Autodesk Fusion 360 part; units mm, degrees
(part 2 of 3)
  spline S18 degree 5 poles (2.4575, 16.735) (2.4592, 16.7471) (2.4624, 16.7712) (2.466, 16.8075) (2.4685, 16.8561) (2.4687, 16.9171) (2.4667, 16.9782) (2.4633, 17.0395) (2.4593, 17.1009) (2.4548, 17.1623) (2.4497, 17.2237) (2.4439, 17.2852) (2.4372, 17.3467) (2.4294, 17.4083) (2.4206, 17.4699) (2.4107, 17.5316) (2.4, 17.5933) (2.3886, 17.6549) (2.3766, 17.7166) (2.364, 17.7783) (2.3508, 17.84) (2.337, 17.9017) (2.3225, 17.9634) (2.3073, 18.025) (2.2914, 18.0867) (2.2749, 18.1483) (2.2578, 18.2099) (2.2401, 18.2715) (2.2219, 18.3331) (2.2031, 18.3946) (2.1837, 18.4561) (2.1638, 18.5175) (2.1433, 18.579) (2.1223, 18.6403) (2.1007, 18.7017) (2.0786, 18.763) (2.056, 18.8242) (2.0329, 18.8854) (2.0092, 18.9465) (1.9851, 19.0076) (1.9605, 19.0686) (1.9353, 19.1296) (1.9097, 19.1905) (1.8836, 19.2514) (1.857, 19.3121) (1.8299, 19.3728) (1.8024, 19.4335) (1.7743, 19.494) (1.7459, 19.5545) (1.7169, 19.615) (1.6875, 19.6753) (1.6577, 19.7355) (1.6274, 19.7957) (1.5966, 19.8558) (1.5654, 19.9158) (1.5338, 19.9757) (1.5017, 20.0356) (1.4692, 20.0953) (1.4362, 20.155) (1.4029, 20.2145) (1.3691, 20.274) (1.3348, 20.3333) (1.3002, 20.3926) (1.2651, 20.4518) (1.2296, 20.5108) (1.1937, 20.5698) (1.1574, 20.6286) (1.1207, 20.6874) (1.0836, 20.746) (1.0461, 20.8045) (1.0082, 20.8629) (0.9775, 20.9095) (0.9544, 20.9445) (0.9388, 20.9677) (0.931, 20.9794) knots 0 0 0 0 0 0 0.01428571 0.02857143 0.04285714 0.05714286 0.07142857 0.08571429 0.1 0.11428571 0.12857143 0.14285714 0.15714286 0.17142857 0.18571429 0.2 0.21428571 0.22857143 0.24285714 0.25714286 0.27142857 0.28571429 0.3 0.31428571 0.32857143 0.34285714 0.35714286 0.37142857 0.38571429 0.4 0.41428571 0.42857143 0.44285714 0.45714286 0.47142857 0.48571429 0.5 0.51428571 0.52857143 0.54285714 0.55714286 0.57142857 0.58571429 0.6 0.61428571 0.62857143 0.64285714 0.65714286 0.67142857 0.68571429 0.7 0.71428571 0.72857143 0.74285714 0.75714286 0.77142857 0.78571429 0.8 0.81428571 0.82857143 0.84285714 0.85714286 0.87142857 0.88571429 0.9 0.91428571 0.92857143 0.94285714 0.95714286 0.97142857 0.98571429 1 1 1 1 1 1
  arc A29 (0.931, 20.9794) -> (-0.931, 20.9794) centre (0, 0) ccw
  spline S19 degree 5 poles (-0.931, 20.9794) (-0.9388, 20.9677) (-0.9544, 20.9445) (-0.9775, 20.9095) (-1.0082, 20.8629) (-1.0461, 20.8045) (-1.0836, 20.746) (-1.1207, 20.6874) (-1.1574, 20.6286) (-1.1937, 20.5698) (-1.2296, 20.5108) (-1.2651, 20.4518) (-1.3002, 20.3926) (-1.3348, 20.3333) (-1.3691, 20.274) (-1.4029, 20.2145) (-1.4362, 20.155) (-1.4692, 20.0953) (-1.5017, 20.0356) (-1.5338, 19.9757) (-1.5654, 19.9158) (-1.5966, 19.8558) (-1.6274, 19.7957) (-1.6577, 19.7355) (-1.6875, 19.6753) (-1.7169, 19.615) (-1.7459, 19.5545) (-1.7743, 19.494) (-1.8024, 19.4335) (-1.8299, 19.3728) (-1.857, 19.3121) (-1.8836, 19.2514) (-1.9097, 19.1905) (-1.9353, 19.1296) (-1.9605, 19.0686) (-1.9851, 19.0076) (-2.0092, 18.9465) (-2.0329, 18.8854) (-2.056, 18.8242) (-2.0786, 18.763) (-2.1007, 18.7017) (-2.1223, 18.6403) (-2.1433, 18.579) (-2.1638, 18.5175) (-2.1837, 18.4561) (-2.2031, 18.3946) (-2.2219, 18.3331) (-2.2401, 18.2715) (-2.2578, 18.2099) (-2.2749, 18.1483) (-2.2914, 18.0867) (-2.3073, 18.025) (-2.3225, 17.9634) (-2.337, 17.9017) (-2.3508, 17.84) (-2.364, 17.7783) (-2.3766, 17.7166) (-2.3886, 17.6549) (-2.4, 17.5933) (-2.4107, 17.5316) (-2.4206, 17.4699) (-2.4294, 17.4083) (-2.4372, 17.3467) (-2.4439, 17.2852) (-2.4497, 17.2237) (-2.4548, 17.1623) (-2.4593, 17.1009) (-2.4633, 17.0395) (-2.4667, 16.9782) (-2.4687, 16.9171) (-2.4685, 16.8561) (-2.466, 16.8075) (-2.4624, 16.7712) (-2.4592, 16.7471) (-2.4575, 16.735) knots -1 -1 -1 -1 -1 -1 -0.98571429 -0.97142857 -0.95714286 -0.94285714 -0.92857143 -0.91428571 -0.9 -0.88571429 -0.87142857 -0.85714286 -0.84285714 -0.82857143 -0.81428571 -0.8 -0.78571429 -0.77142857 -0.75714286 -0.74285714 -0.72857143 -0.71428571 -0.7 -0.68571429 -0.67142857 -0.65714286 -0.64285714 -0.62857143 -0.61428571 -0.6 -0.58571429 -0.57142857 -0.55714286 -0.54285714 -0.52857143 -0.51428571 -0.5 -0.48571429 -0.47142857 -0.45714286 -0.44285714 -0.42857143 -0.41428571 -0.4 -0.38571429 -0.37142857 -0.35714286 -0.34285714 -0.32857143 -0.31428571 -0.3 -0.28571429 -0.27142857 -0.25714286 -0.24285714 -0.22857143 -0.21428571 -0.2 -0.18571429 -0.17142857 -0.15714286 -0.14285714 -0.12857143 -0.11428571 -0.1 -0.08571429 -0.07142857 -0.05714286 -0.04285714 -0.02857143 -0.01428571 0 0 0 0 0 0
  line L19 (-2.4575, 16.735) -> (-2.2515, 15.3323)
  arc A30 (-3.0322, 14.2091) -> (-2.2515, 15.3323) centre (-3.2409, 15.1871) ccw
  arc A31 (-5.7163, 14.4039) -> (-4.4786, 13.8215) centre (-4.7868, 14.7728) ccw
  line L20 (-5.7163, 14.4039) -> (-6.2393, 15.7217)
  spline S20 degree 5 poles (-6.2393, 15.7217) (-6.2438, 15.733) (-6.2531, 15.7555) (-6.2682, 15.7887) (-6.2903, 15.8321) (-6.3206, 15.885) (-6.3529, 15.9369) (-6.3864, 15.9883) (-6.4206, 16.0394) (-6.4553, 16.0903) (-6.4904, 16.141) (-6.5261, 16.1914) (-6.5627, 16.2413) (-6.6002, 16.2907) (-6.6387, 16.3397) (-6.678, 16.3882) (-6.7181, 16.4362) (-6.7588, 16.4839) (-6.8001, 16.5314) (-6.8418, 16.5785) (-6.8841, 16.6253) (-6.927, 16.6718) (-6.9703, 16.718) (-7.0143, 16.7638) (-7.0589, 16.8092) (-7.104, 16.8544) (-7.1496, 16.8992) (-7.1957, 16.9436) (-7.2423, 16.9878) (-7.2894, 17.0317) (-7.3369, 17.0753) (-7.3849, 17.1185) (-7.4333, 17.1615) (-7.4822, 17.2042) (-7.5315, 17.2465) (-7.5813, 17.2885) (-7.6315, 17.3303) (-7.6822, 17.3717) (-7.7332, 17.4128) (-7.7847, 17.4536) (-7.8365, 17.4942) (-7.8888, 17.5344) (-7.9414, 17.5743) (-7.9944, 17.614) (-8.0479, 17.6533) (-8.1017, 17.6923) (-8.1559, 17.7311) (-8.2104, 17.7695) (-8.2653, 17.8077) (-8.3206, 17.8455) (-8.3762, 17.8831) (-8.4322, 17.9203) (-8.4885, 17.9573) (-8.5452, 17.9939) (-8.6022, 18.0303) (-8.6596, 18.0664) (-8.7173, 18.1022) (-8.7753, 18.1376) (-8.8337, 18.1728) (-8.8924, 18.2077) (-8.9514, 18.2423) (-9.0107, 18.2766) (-9.0703, 18.3106) (-9.1303, 18.3443) (-9.1905, 18.3777) (-9.2511, 18.4108) (-9.3119, 18.4436) (-9.3731, 18.4761) (-9.4345, 18.5084) (-9.4963, 18.5403) (-9.5583, 18.5719) (-9.6082, 18.597) (-9.6457, 18.6156) (-9.6708, 18.628) (-9.6834, 18.6342) knots 0 0 0 0 0 0 0.01428571 0.02857143 0.04285714 0.05714286 0.07142857 0.08571429 0.1 0.11428571 0.12857143 0.14285714 0.15714286 0.17142857 0.18571429 0.2 0.21428571 0.22857143 0.24285714 0.25714286 0.27142857 0.28571429 0.3 0.31428571 0.32857143 0.34285714 0.35714286 0.37142857 0.38571429 0.4 0.41428571 0.42857143 0.44285714 0.45714286 0.47142857 0.48571429 0.5 0.51428571 0.52857143 0.54285714 0.55714286 0.57142857 0.58571429 0.6 0.61428571 0.62857143 0.64285714 0.65714286 0.67142857 0.68571429 0.7 0.71428571 0.72857143 0.74285714 0.75714286 0.77142857 0.78571429 0.8 0.81428571 0.82857143 0.84285714 0.85714286 0.87142857 0.88571429 0.9 0.91428571 0.92857143 0.94285714 0.95714286 0.97142857 0.98571429 1 1 1 1 1 1
  arc A32 (-9.6834, 18.6342) -> (-11.296, 17.7031) centre (0, 0) ccw
  spline S21 degree 5 poles (-11.296, 17.7031) (-11.2969, 17.6892) (-11.2987, 17.6613) (-11.3013, 17.6194) (-11.3046, 17.5637) (-11.3082, 17.4942) (-11.3114, 17.4247) (-11.3143, 17.3554) (-11.3167, 17.2862) (-11.3187, 17.2171) (-11.3203, 17.1481) (-11.3215, 17.0792) (-11.3223, 17.0104) (-11.3227, 16.9418) (-11.3226, 16.8733) (-11.3222, 16.8049) (-11.3213, 16.7366) (-11.32, 16.6685) (-11.3183, 16.6005) (-11.3161, 16.5326) (-11.3136, 16.4649) (-11.3106, 16.3973) (-11.3072, 16.3299) (-11.3033, 16.2627) (-11.2991, 16.1955) (-11.2944, 16.1286) (-11.2892, 16.0618) (-11.2836, 15.9952) (-11.2776, 15.9287) (-11.2712, 15.8624) (-11.2643, 15.7963) (-11.2569, 15.7304) (-11.2491, 15.6646) (-11.2408, 15.5991) (-11.2321, 15.5337) (-11.223, 15.4685) (-11.2133, 15.4036) (-11.2032, 15.3388) (-11.1927, 15.2742) (-11.1816, 15.2099) (-11.1701, 15.1458) (-11.1581, 15.0819) (-11.1456, 15.0182) (-11.1327, 14.9548) (-11.1192, 14.8916) (-11.1052, 14.8286) (-11.0907, 14.766) (-11.0758, 14.7035) (-11.0603, 14.6413) (-11.0443, 14.5794) (-11.0278, 14.5178) (-11.0107, 14.4565) (-10.993, 14.3955) (-10.9747, 14.3348) (-10.9559, 14.2745) (-10.9365, 14.2145) (-10.9165, 14.1547) (-10.8961, 14.0953) (-10.8751, 14.0362) (-10.8535, 13.9774) (-10.8312, 13.9191) (-10.8081, 13.8613) (-10.7841, 13.8041) (-10.7591, 13.7475) (-10.7334, 13.6913) (-10.707, 13.6356) (-10.6803, 13.5801) (-10.6531, 13.525) (-10.6253, 13.4703) (-10.5965, 13.4163) (-10.5658, 13.3636) (-10.5393, 13.3228) (-10.5181, 13.2931) (-10.5033, 13.2738) (-10.4957, 13.2642) knots -1 -1 -1 -1 -1 -1 -0.98571429 -0.97142857 -0.95714286 -0.94285714 -0.92857143 -0.91428571 -0.9 -0.88571429 -0.87142857 -0.85714286 -0.84285714 -0.82857143 -0.81428571 -0.8 -0.78571429 -0.77142857 -0.75714286 -0.74285714 -0.72857143 -0.71428571 -0.7 -0.68571429 -0.67142857 -0.65714286 -0.64285714 -0.62857143 -0.61428571 -0.6 -0.58571429 -0.57142857 -0.55714286 -0.54285714 -0.52857143 -0.51428571 -0.5 -0.48571429 -0.47142857 -0.45714286 -0.44285714 -0.42857143 -0.41428571 -0.4 -0.38571429 -0.37142857 -0.35714286 -0.34285714 -0.32857143 -0.31428571 -0.3 -0.28571429 -0.27142857 -0.25714286 -0.24285714 -0.22857143 -0.21428571 -0.2 -0.18571429 -0.17142857 -0.15714286 -0.14285714 -0.12857143 -0.11428571 -0.1 -0.08571429 -0.07142857 -0.05714286 -0.04285714 -0.02857143 -0.01428571 0 0 0 0 0 0
  line L21 (-10.4957, 13.2642) -> (-9.616, 12.1524)
  arc A33 (-9.7305, 10.7893) -> (-9.616, 12.1524) centre (-10.4002, 11.5319) ccw
  arc A34 (-12.1524, 9.616) -> (-10.7893, 9.7305) centre (-11.5319, 10.4002) ccw
  line L22 (-12.1524, 9.616) -> (-13.2642, 10.4957)
  spline S22 degree 5 poles (-13.2642, 10.4957) (-13.2738, 10.5033) (-13.2931, 10.5181) (-13.3228, 10.5393) (-13.3636, 10.5658) (-13.4163, 10.5965) (-13.4703, 10.6253) (-13.525, 10.6531) (-13.5801, 10.6803) (-13.6356, 10.707) (-13.6913, 10.7334) (-13.7475, 10.7591) (-13.8041, 10.7841) (-13.8613, 10.8081) (-13.9191, 10.8312) (-13.9774, 10.8535) (-14.0362, 10.8751) (-14.0953, 10.8961) (-14.1547, 10.9165) (-14.2145, 10.9365) (-14.2745, 10.9559) (-14.3348, 10.9747) (-14.3955, 10.993) (-14.4565, 11.0107) (-14.5178, 11.0278) (-14.5794, 11.0443) (-14.6413, 11.0603) (-14.7035, 11.0758) (-14.766, 11.0907) (-14.8286, 11.1052) (-14.8916, 11.1192) (-14.9548, 11.1327) (-15.0182, 11.1456) (-15.0819, 11.1581) (-15.1458, 11.1701) (-15.2099, 11.1816) (-15.2742, 11.1927) (-15.3388, 11.2032) (-15.4036, 11.2133) (-15.4685, 11.223) (-15.5337, 11.2321) (-15.5991, 11.2408) (-15.6646, 11.2491) (-15.7304, 11.2569) (-15.7963, 11.2643) (-15.8624, 11.2712) (-15.9287, 11.2776) (-15.9952, 11.2836) (-16.0618, 11.2892) (-16.1286, 11.2944) (-16.1955, 11.2991) (-16.2627, 11.3033) (-16.3299, 11.3072) (-16.3973, 11.3106) (-16.4649, 11.3136) (-16.5326, 11.3161) (-16.6005, 11.3183) (-16.6685, 11.32) (-16.7366, 11.3213) (-16.8049, 11.3222) (-16.8733, 11.3226) (-16.9418, 11.3227) (-17.0104, 11.3223) (-17.0792, 11.3215) (-17.1481, 11.3203) (-17.2171, 11.3187) (-17.2862, 11.3167) (-17.3554, 11.3143) (-17.4247, 11.3114) (-17.4942, 11.3082) (-17.5637, 11.3046) (-17.6194, 11.3013) (-17.6613, 11.2987) (-17.6892, 11.2969) (-17.7031, 11.296) knots 0 0 0 0 0 0 0.01428571 0.02857143 0.04285714 0.05714286 0.07142857 0.08571429 0.1 0.11428571 0.12857143 0.14285714 0.15714286 0.17142857 0.18571429 0.2 0.21428571 0.22857143 0.24285714 0.25714286 0.27142857 0.28571429 0.3 0.31428571 0.32857143 0.34285714 0.35714286 0.37142857 0.38571429 0.4 0.41428571 0.42857143 0.44285714 0.45714286 0.47142857 0.48571429 0.5 0.51428571 0.52857143 0.54285714 0.55714286 0.57142857 0.58571429 0.6 0.61428571 0.62857143 0.64285714 0.65714286 0.67142857 0.68571429 0.7 0.71428571 0.72857143 0.74285714 0.75714286 0.77142857 0.78571429 0.8 0.81428571 0.82857143 0.84285714 0.85714286 0.87142857 0.88571429 0.9 0.91428571 0.92857143 0.94285714 0.95714286 0.97142857 0.98571429 1 1 1 1 1 1
  arc A35 (-17.7031, 11.296) -> (-18.6342, 9.6834) centre (0, 0) ccw
  spline S23 degree 5 poles (-18.6342, 9.6834) (-18.628, 9.6708) (-18.6156, 9.6457) (-18.597, 9.6082) (-18.5719, 9.5583) (-18.5403, 9.4963) (-18.5084, 9.4345) (-18.4761, 9.3731) (-18.4436, 9.3119) (-18.4108, 9.2511) (-18.3777, 9.1905) (-18.3443, 9.1303) (-18.3106, 9.0703) (-18.2766, 9.0107) (-18.2423, 8.9514) (-18.2077, 8.8924) (-18.1728, 8.8337) (-18.1376, 8.7753) (-18.1022, 8.7173) (-18.0664, 8.6596) (-18.0303, 8.6022) (-17.9939, 8.5452) (-17.9573, 8.4885) (-17.9203, 8.4322) (-17.8831, 8.3762) (-17.8455, 8.3206) (-17.8077, 8.2653) (-17.7695, 8.2104) (-17.7311, 8.1559) (-17.6923, 8.1017) (-17.6533, 8.0479) (-17.614, 7.9944) (-17.5743, 7.9414) (-17.5344, 7.8888) (-17.4942, 7.8365) (-17.4536, 7.7847) (-17.4128, 7.7332) (-17.3717, 7.6822) (-17.3303, 7.6315) (-17.2885, 7.5813) (-17.2465, 7.5315) (-17.2042, 7.4822) (-17.1615, 7.4333) (-17.1185, 7.3849) (-17.0753, 7.3369) (-17.0317, 7.2894) (-16.9878, 7.2423) (-16.9436, 7.1957) (-16.8992, 7.1496) (-16.8544, 7.104) (-16.8092, 7.0589) (-16.7638, 7.0143) (-16.718, 6.9703) (-16.6718, 6.927) (-16.6253, 6.8841) (-16.5785, 6.8418) (-16.5314, 6.8001) (-16.4839, 6.7588) (-16.4362, 6.7181) (-16.3882, 6.678) (-16.3397, 6.6387) (-16.2907, 6.6002) (-16.2413, 6.5627) (-16.1914, 6.5261) (-16.141, 6.4904) (-16.0903, 6.4553) (-16.0394, 6.4206) (-15.9883, 6.3864) (-15.9369, 6.3529) (-15.885, 6.3206) (-15.8321, 6.2903) (-15.7887, 6.2682) (-15.7555, 6.2531) (-15.733, 6.2438) (-15.7217, 6.2393) knots -1 -1 -1 -1 -1 -1 -0.98571429 -0.97142857 -0.95714286 -0.94285714 -0.92857143 -0.91428571 -0.9 -0.88571429 -0.87142857 -0.85714286 -0.84285714 -0.82857143 -0.81428571 -0.8 -0.78571429 -0.77142857 -0.75714286 -0.74285714 -0.72857143 -0.71428571 -0.7 -0.68571429 -0.67142857 -0.65714286 -0.64285714 -0.62857143 -0.61428571 -0.6 -0.58571429 -0.57142857 -0.55714286 -0.54285714 -0.52857143 -0.51428571 -0.5 -0.48571429 -0.47142857 -0.45714286 -0.44285714 -0.42857143 -0.41428571 -0.4 -0.38571429 -0.37142857 -0.35714286 -0.34285714 -0.32857143 -0.31428571 -0.3 -0.28571429 -0.27142857 -0.25714286 -0.24285714 -0.22857143 -0.21428571 -0.2 -0.18571429 -0.17142857 -0.15714286 -0.14285714 -0.12857143 -0.11428571 -0.1 -0.08571429 -0.07142857 -0.05714286 -0.04285714 -0.02857143 -0.01428571 0 0 0 0 0 0
  line L23 (-15.7217, 6.2393) -> (-14.4039, 5.7163)
  arc A36 (-13.8215, 4.4786) -> (-14.4039, 5.7163) centre (-14.7728, 4.7868) ccw
  circle A37 centre (0, 0) radius 10 construction
  circle A38 centre (-10, 0) radius 2
  arc A39 (-14.2091, -3.0322) -> (-13.8215, -4.4786) centre (0, 0) ccw
  arc A40 (-10.7893, -9.7305) -> (-9.7305, -10.7893) centre (0, 0) ccw
  arc A41 (-4.4786, -13.8215) -> (-3.0322, -14.2091) centre (0, 0) ccw
  arc A42 (3.0322, -14.2091) -> (4.4786, -13.8215) centre (0, 0) ccw
  arc A43 (9.7305, -10.7893) -> (10.7893, -9.7305) centre (0, 0) ccw
  arc A44 (13.8215, -4.4786) -> (14.2091, -3.0322) centre (0, 0) ccw
  arc A45 (14.2091, 3.0322) -> (13.8215, 4.4786) centre (0, 0) ccw
  arc A46 (10.7893, 9.7305) -> (9.7305, 10.7893) centre (0, 0) ccw
  arc A47 (4.4786, 13.8215) -> (3.0322, 14.2091) centre (0, 0) ccw
  arc A48 (-3.0322, 14.2091) -> (-4.4786, 13.8215) centre (0, 0) ccw
  arc A49 (-9.7305, 10.7893) -> (-10.7893, 9.7305) centre (0, 0) ccw
  circle A50 centre (0, 0) radius 1.75
  circle A51 centre (0, 0) radius 3.5
  line L24 (-10, -4) -> (30, -4)
  arc A52 (30, -4) -> (30, 4) centre (30, 0) ccw
  line L25 (30, 4) -> (-10, 4)
  arc A53 (-10, 4) -> (-10, -4) centre (-10, 0) ccw
  line L26 (-10, 0) -> (30, 0) construction
  circle A54 centre (30, 0) radius 2
  dimension "d15" = 20
  dimension "d16" = 4
  dimension "d25" = 7
  dimension "d27" = 8
  dimension "d28" = 4
  constraint coincident A0.centre A2.centre
  constraint coincident A37 A38.centre
  constraint tangent L24 A52
  constraint tangent A52 L25
  constraint parallel L24 L25
  constraint tangent L25 A53
  constraint tangent L24 A53
  constraint horizontal L26
  constraint coincident A38.centre A53.centre
  constraint concentric A52 A54
  measures "d15" diameter of A37
  measures "d16" diameter of A38
  measures "d25" diameter of A51
  measures "d27" diameter of A52
  measures "d28" diameter of A54
extrude "Extrude4" add sketch "Connecting Rod" along normal blind 5 separate body contours A19 L12 S12 A20 S13 L13 A21 A44 A45 L24 A52 L25 | A19 L12 S12 A20 S13 L13 A21 A44 A45 L24 L25 A53 | A50 | A51 makes body 2
extrude "Extrude5" cut sketch "Connecting Rod" against normal blind 2 contours A51 bodies 1
sketch "Slider" plane through (0, 0, 7) normal (0, 0, 1) x (-1, 0, 0)
  line L0 (26, 5) -> (46, 5)
  line L1 (46, 5) -> (46, -5)
  line L2 (46, -5) -> (26, -5)
  line L3 (26, -5) -> (26, 5)
  circle A0 centre (30, 0) radius 2
  dimension "d33" = 10
  dimension "d34" = 20
  constraint horizontal L0
  constraint vertical L1
  constraint horizontal L2
  constraint vertical L3
  measures "d33" distance of L0.end L1.end
  measures "d34" distance of L0.start L0.end
extrude "Extrude6" add sketch "Slider" against normal blind 7 separate body makes body 3
extrude "Extrude7" add sketch "Connecting Rod" against normal blind 7 contours A54 bodies 3
extrude "Extrude8" add sketch "Connecting Rod" along normal blind 5 contours A38 bodies 1
extrude "Extrude9" add sketch "Connecting Rod" along normal blind 5 contours A54 bodies 3
sketch "Slider Dowel Hole" plane through (-46, 0, 0) normal (-1, 0, 0) x (0, -1, 0)
  line L0 (5, 7) -> (-5, 7)
  line L1 (-5, 7) -> (-5, 0)
  line L2 (-5, 0) -> (5, 0)
  line L3 (5, 0) -> (5, 7)
  line L4 (0, 1.75) -> (0, 22.5)
  circle A0 centre (0, 3.5) radius 2.75
  point P0 (2.2515, 7)
  dimension "d44" = 5.5
  dimension "d45" = 3.5
  constraint coincident L4 A0.centre
  measures "d44" diameter of A0
  measures "d45" vertical distance of A0.centre P0
extrude "Extrude10" cut sketch "Slider Dowel Hole" against normal blind 15 contours A0 bodies 3
sketch "Base Plate" plane through (0, 0, 0) normal (0, 0, 1) x (1, 0, 0)
  line L0 (42, -25) -> (-86, -25) construction
  line L1 (-86, -25) -> (-86, 25) construction
  line L2 (-86, 25) -> (42, 25) construction
  line L3 (42, 25) -> (42, -25) construction
  line L4 (-46, -5) -> (-46, 5)
  line L5 (0, 0) -> (27, 0) construction
  circle A0 centre (27, 0) radius 1.5
  circle A1 centre (0, 0) radius 1.5
  line L6 (-23.5, -5.3) -> (-83.5, -5.3)
  line L7 (-83.5, -5.3) -> (-83.5, -10.3)
  line L8 (-83.5, -10.3) -> (-23.5, -10.3)
  line L9 (-23.5, -10.3) -> (-23.5, -5.3)
  line L10 (-26, -5) -> (-46, -5)
  line L11 (-26, 5) -> (-26, -5)
  line L12 (-23.5, 5.3) -> (-83.5, 5.3)
  line L13 (-83.5, 5.3) -> (-83.5, 10.3)
  line L14 (-83.5, 10.3) -> (-23.5, 10.3)
  line L15 (-23.5, 10.3) -> (-23.5, 5.3)
  line L16 (-89, -16) -> (-86, -16)
  line L17 (-86, -8) -> (-89, -8)
  line L18 (-89, -8) -> (-89, -16)
  line L19 (-86, 0) -> (-102, 0) construction
  line L20 (-86, -25) -> (-86, -16) construction
  line L21 (-86, -25) -> (-86, -16) construction
  line L22 (-86, -25) -> (-86, -16)
  line L23 (-86, -8) -> (-86, 0)
  line L24 (-86, 8) -> (-89, 8)
  line L25 (-89, 8) -> (-89, 16)
  line L26 (-89, 16) -> (-86, 16)
  line L27 (-86, 25) -> (-86, 16)
  line L28 (-86, 8) -> (-86, 0)
  line L29 (-66, 28) -> (-54, 28)
  line L30 (-54, 28) -> (-54, 25)
  line L31 (-66, 25) -> (-66, 28)
  line L32 (-86, 25) -> (-66, 25)
  line L33 (-54, 25) -> (-34, 25)
  line L34 (-34, 25) -> (-34, 28)
  line L35 (-34, 28) -> (-22, 28)
  line L36 (-22, 28) -> (-22, 25)
  line L37 (-22, 25) -> (-2, 25)
  line L38 (-2, 25) -> (-2, 28)
  line L39 (-2, 28) -> (10, 28)
  line L40 (10, 28) -> (10, 25)
  line L41 (10, 25) -> (30, 25)
  line L42 (30, 25) -> (30, 28)
  line L43 (30, 28) -> (42, 28)
  line L44 (42, 28) -> (42, 25)
  line L45 (-22, 25) -> (-22, -25) construction
  line L46 (42, 25) -> (42, 16)
  line L47 (45, 16) -> (42, 16)
  line L48 (45, 8) -> (45, 16)
  line L49 (42, 8) -> (45, 8)
  line L50 (42, 8) -> (42, 0)
  line L51 (42, -8) -> (42, 0)
  line L52 (42, -8) -> (45, -8)
  line L53 (45, -8) -> (45, -16)
  line L54 (45, -16) -> (42, -16)
  line L55 (42, -25) -> (42, -16)
  line L56 (10, 0) -> (-30, 0) construction
  line L57 (-66, -28) -> (-54, -28)
  line L58 (-66, -25) -> (-66, -28)
  line L59 (10, -28) -> (10, -25)
  line L60 (-2, -25) -> (-2, -28)
  line L61 (-2, -28) -> (10, -28)
  line L62 (-34, -25) -> (-34, -28)
  line L63 (-86, -25) -> (-66, -25)
  line L64 (10, -25) -> (30, -25)
  line L65 (42, -28) -> (42, -25)
  line L66 (30, -25) -> (30, -28)
  line L67 (-22, -28) -> (-22, -25)
  line L68 (-54, -25) -> (-34, -25)
  line L69 (-34, -28) -> (-22, -28)
  line L70 (30, -28) -> (42, -28)
  line L71 (-54, -28) -> (-54, -25)
  line L72 (-22, -25) -> (-2, -25)
  point P0 (42, -25)
  point P1 (-86, -25)
  point P2 (42, -25)
  dimension "d48" = 25
  dimension "d49" = 50
  dimension "d50" = 40
  dimension "d51" = 27
  dimension "d52" = 3
  dimension "d53" = 3
  dimension "d54" = 15
  dimension "d55" = 0.3
  dimension "d57" = 2.5
  dimension "d58" = 60
  dimension "d59" = 5
  dimension "d64" = 3
  dimension "d65" = 8
  dimension "d66" = 8
  dimension "d67" = 9
  dimension "d68" = 12
  dimension "d69" = 3
  dimension "d70" = 20
  dimension "d73" = 96
  dimension "d74" = 0
  dimension "d82" = 128
  constraint horizontal L0
  constraint vertical L1
  constraint horizontal L2
  constraint vertical L3
  constraint coincident L5.start A1.centre
  constraint horizontal L5
  constraint coincident L5.end A0.centre
  constraint horizontal L6
  constraint vertical L7
  constraint horizontal L8
  constraint vertical L9
  constraint symmetric L5 L6.start L12.start
  constraint symmetric L5 L6.end L12.end
  constraint symmetric L5 L7.end L13.end
  constraint symmetric L5 L8.end L14.end
  constraint horizontal L16
  constraint horizontal L17
  constraint vertical L18
  constraint coincident L1 L17.start
  constraint midpoint L1 L19.start
  constraint perpendicular L1 L19
  constraint symmetric P1 L19 L1.end
  constraint symmetric L16.start L19 L25.end
  constraint symmetric L16.end L19 L26.end
  constraint symmetric L17.start L19 L24.start
  constraint symmetric L17.end L19 L24.end
  constraint symmetric L23.end L19 L28.end
  constraint horizontal L29
  constraint vertical L30
  constraint vertical L31
  constraint coincident L2 L30.end
  constraint midpoint L0 L45.end
  constraint symmetric P1 L45 P0
  constraint symmetric L16.start L45 L53.end
  constraint symmetric L16.end L45 L54.end
  constraint symmetric L17.start L45 L51.start
  constraint symmetric L17.end L45 L52.end
  constraint symmetric L19.start L45 L50.end
  constraint symmetric L24.start L45 L49.start
  constraint symmetric L24.end L45 L48.start
  constraint symmetric L25.end L45 L47.start
  constraint symmetric L26.end L45 L46.end
  constraint symmetric L1.end L45 L2.end
  constraint symmetric L1.end L56 P1
  constraint symmetric L2.end L56 P2
  constraint symmetric L29.start L56 L57.start
  constraint symmetric L29.end L56 L57.end
  constraint symmetric L30.end L56 L68.start
  constraint symmetric L31.start L56 L58.start
  constraint symmetric L33.end L56 L62.start
  constraint symmetric L34.end L56 L62.end
  constraint symmetric L35.end L56 L67.start
  constraint symmetric L36.end L56 L45.end
  constraint symmetric L37.end L56 L60.start
  constraint symmetric L38.end L56 L60.end
  constraint symmetric L39.end L56 L59.start
  constraint symmetric L40.end L56 L59.end
  constraint symmetric L41.end L56 L64.end
  constraint symmetric L42.end L56 L66.end
  constraint symmetric L43.end L56 L65.start
  measures "d48" distance of L0 L5.start
  measures "d49" distance of P2 L2.end
  measures "d50" distance of L1 L4
  measures "d51" distance of L5.start L5.end
  measures "d52" diameter of A0
  measures "d53" diameter of A1
  measures "d54" distance of L3 L5.end
  measures "d55" distance of L6 L10
  measures "d57" distance of L9 L11
  measures "d58" distance of L7.end L8.end
  measures "d59" distance of L6.end L7.end
  measures "d64" distance of L17.start L17.end
  measures "d65" distance of L16.start L17.end
  measures "d66" distance of L17 L19
  measures "d67" distance of P1 L16.end
  measures "d68" distance of L29.start L29.end
  measures "d69" distance of L29.start L31.start
  measures "d70" distance of L27 L31
  measures "d82" distance of L1.end L2.end
extrude "Extrude11" add sketch "Base Plate" along normal blind 6.7 separate body contours L6 L7 L8 L9 | L12 L13 L14 L15 makes body 4 at (-63.5, -10.3, 2.2333) makes body 5 at (-43.5, 5.3, 2.2333)
extrude "Extrude12" add sketch "Base Plate" against normal blind 3 separate body contours L6 L7 L8 L9 | L12 L13 L14 L15 | L16 L17 L18 L22 L23 L24 L25 L26 L27 L28 L29 L30 L31 L32 L33 L34 L35 L36 L37 L38 L39 L40 L41 L42 L43 L44 L46 L47 L48 L49 L50 L51 L52 L53 L54 L55 L57 L58 L59 L60 L61 L62 L63 L64 L65 L66 L67 L68 L69 L70 L71 L72 makes body 6
combine "Combine1" operation add target body 4 tool bodies 5 6
sketch "Top Plate" plane through (-86, 0, 0) normal (-1, 0, 0) x (0, -1, 0)
  line L0 (0, 0) -> (-8, 0)
  line L1 (-8, 0) -> (-8, -3)
  line L2 (-8, -3) -> (0, -3)
  line L3 (0, -3) -> (0, 0)
  line L4 (-16, 0) -> (-16, -3)
  line L5 (-8, 0) -> (-16, 0)
  line L6 (-8, 0) -> (-16, 0)
  line L7 (-16, 0) -> (-16, -3)
  line L8 (-16, -3) -> (-8, -3)
  line L9 (-8, -3) -> (-8, 0)
  line L10 (-8, 0) -> (-8, -3)
  line L11 (-8, -3) -> (-16, -3)
  line L12 (8, 0) -> (8, -3)
  line L13 (8, 0) -> (16, 0)
  line L14 (16, 0) -> (8, 0)
  line L15 (8, 0) -> (8, -3)
  line L16 (8, -3) -> (16, -3)
  line L17 (16, -3) -> (16, 0)
  line L18 (16, 0) -> (16, -3)
  line L19 (16, -3) -> (8, -3)
  circle A0 centre (0, 3.5) radius 2.75
  line L20 (0, 3.5) -> (0, 23.5) construction
  circle A1 centre (0, 23.5) radius 2.75
  line L21 (0, 3.5) -> (25, 3.5) construction
  circle A2 centre (0, -16.5) radius 2.75
  circle A3 centre (0, 23.5) radius 4.75
  circle A4 centre (0, -16.5) radius 4.75
  line L22 (-25, -25) -> (-25, 49) construction
  line L23 (-25, 49) -> (25, 49) construction
  line L24 (25, 49) -> (25, -25) construction
  line L25 (-17.7031, 7) -> (-13.2642, 7)
  line L26 (25, 12) -> (-25, 12) construction
  line L27 (25, -19) -> (28, -19)
  line L28 (28, -19) -> (28, -9)
  line L29 (28, -9) -> (25, -9)
  line L30 (25, 12) -> (28, 12)
  line L31 (28, 12) -> (28, 22)
  line L32 (28, 22) -> (25, 22)
  line L33 (25, 30) -> (28, 30)
  line L34 (28, 30) -> (28, 40)
  line L35 (28, 40) -> (25, 40)
  line L36 (9, 49) -> (9, 52)
  line L37 (9, 52) -> (17, 52)
  line L38 (17, 52) -> (17, 49)
  line L39 (25, 49) -> (25, 40)
  line L40 (25, 30) -> (25, 22)
  line L41 (25, 12) -> (25, -9)
  line L42 (25, -19) -> (25, -25)
  line L43 (25, 49) -> (17, 49)
  line L44 (9, 49) -> (0, 49)
  line L45 (-25, 30) -> (-25, 22)
  line L46 (-28, 40) -> (-25, 40)
  line L47 (-28, -19) -> (-28, -9)
  line L48 (-25, -19) -> (-25, -25)
  line L49 (-25, -19) -> (-28, -19)
  line L50 (-28, -9) -> (-25, -9)
  line L51 (-25, 49) -> (-25, 40)
  line L52 (-28, 30) -> (-28, 40)
  line L53 (-25, 12) -> (-25, -9)
  line L54 (-25, 12) -> (-28, 12)
  line L55 (-28, 12) -> (-28, 22)
  line L56 (-28, 22) -> (-25, 22)
  line L57 (-25, 30) -> (-28, 30)
  line L58 (-17, 52) -> (-17, 49)
  line L59 (-9, 49) -> (0, 49)
  line L60 (-9, 52) -> (-17, 52)
  line L61 (-9, 49) -> (-9, 52)
  line L62 (-25, 49) -> (-17, 49)
  line L63 (-25, -25) -> (-17, -25)
  line L64 (9, -28) -> (17, -28)
  line L65 (9, -25) -> (0, -25)
  line L66 (-17, -28) -> (-17, -25)
  line L67 (-9, -25) -> (-9, -28)
  line L68 (9, -25) -> (9, -28)
  line L69 (-9, -25) -> (0, -25)
  line L70 (17, -28) -> (17, -25)
  line L71 (-9, -28) -> (-17, -28)
  line L72 (25, -25) -> (17, -25)
  line L73 (16, -3) -> (8, 0) construction
  line L74 (8, -3) -> (16, 0) construction
  line L75 (7.75, -3.25) -> (16.25, -3.25)
  line L76 (16.25, -3.25) -> (16.25, 0.25)
  line L77 (16.25, 0.25) -> (7.75, 0.25)
  line L78 (7.75, 0.25) -> (7.75, -3.25)
  line L79 (7.75, -3.25) -> (16.25, 0.25) construction
  line L80 (16.25, -3.25) -> (7.75, 0.25) construction
  line L81 (-8, -3) -> (-16, 0) construction
  line L82 (-16, -3) -> (-8, 0) construction
  line L83 (-16.25, -3.25) -> (-7.75, -3.25)
  line L84 (-7.75, -3.25) -> (-7.75, 0.25)
  line L85 (-7.75, 0.25) -> (-16.25, 0.25)
  line L86 (-16.25, 0.25) -> (-16.25, -3.25)
  line L87 (-16.25, -3.25) -> (-7.75, 0.25) construction
  line L88 (-7.75, -3.25) -> (-16.25, 0.25) construction
  point P0 (0, 3.5)
  point P1 (-25, 3.5)
  point P2 (-25, -25)
  point P3 (-25, -25)
  point P4 (12, -1.5)
  point P5 (-12, -1.5)
  dimension "d75" = 20
  dimension "d77" = 5.5
  dimension "d94" = 9.5
  dimension "d95" = 9.5
  dimension "d130" = 50
  dimension "d132" = 42
  dimension "d133" = 10
  dimension "d134" = 3
  dimension "d135" = 10
  dimension "d136" = 3
  dimension "d137" = 3
  dimension "d138" = 10
  dimension "d139" = 8
  dimension "d140" = 3
  dimension "d141" = 8
  dimension "d178" = 8.5
  dimension "d179" = 3.5
  dimension "d180" = 8.5
  dimension "d181" = 3.5
  constraint coincident P0 A0.centre
  constraint vertical L20
  constraint coincident L20.end A1.centre
  constraint symmetric A1 L21 A2
  constraint concentric A2 A4
  constraint vertical L22
  constraint horizontal L23
  constraint vertical L24
  constraint midpoint L24 L26.start
  constraint midpoint L22 L26.end
  constraint horizontal L27
  constraint vertical L28
  constraint horizontal L29
  constraint coincident L24 L27.start
  constraint horizontal L30
  constraint vertical L31
  constraint horizontal L32
  constraint horizontal L33
  constraint vertical L34
  constraint horizontal L35
  constraint coincident L24 L33.start
  constraint vertical L36
  constraint horizontal L37
  constraint vertical L38
  constraint coincident L23 L38.end
  constraint midpoint L23 L44.end
  constraint symmetric L20 L21.end P1
  constraint symmetric L20 L24.end P3
  constraint symmetric L20 L23.end L22.end
  constraint symmetric L20 L26.start L26.end
  constraint symmetric L20 L27.start L48.start
  constraint symmetric L20 L27.end L47.start
  constraint symmetric L20 L28.end L47.end
  constraint symmetric L20 L29.end L50.end
  constraint symmetric L20 L30.end L54.end
  constraint symmetric L20 L31.end L55.end
  constraint symmetric L20 L32.end L45.end
  constraint symmetric L20 L33.start L45.start
  constraint symmetric L20 L33.end L52.start
  constraint symmetric L20 L34.end L46.start
  constraint symmetric L20 L35.end L46.end
  constraint symmetric L20 L38.end L58.end
  constraint symmetric L20 L36.start L59.start
  constraint symmetric L20 L36.end L60.start
  constraint symmetric L20 L37.end L58.start
  constraint symmetric L20 L44.end L59.end
  constraint symmetric L22.end L26 P3
  constraint symmetric L23.end L26 L24.end
  constraint symmetric L26 L38.end L70.end
  constraint symmetric L26 L36.start L65.start
  constraint symmetric L26 L36.end L64.start
  constraint symmetric L26 L37.end L64.end
  constraint symmetric L26 L44.end L65.end
  constraint symmetric L26 L22.end P3
  constraint symmetric L26 L58.start L66.start
  constraint symmetric L26 L58.end L63.end
  constraint symmetric L26 L59.start L67.start
  constraint symmetric L26 L60.start L67.end
  constraint horizontal P0 L21.end
  constraint coincident P3 P2
  constraint coincident L26.end L53.start
  constraint coincident L65.end L69.end
  constraint coincident L24.end L42.end
  constraint parallel L22 L53
  constraint parallel L51 L66
  constraint parallel L60 L69
  constraint parallel L45 L51
  constraint vertical L21.end L24.end
  constraint equal L0 L40
  constraint coincident L16.end L17.start
  constraint coincident L12.start L13.start
  constraint coincident L12.end L15.end
  constraint coincident L13.end L14.start
  constraint horizontal L75
  constraint perpendicular L75 L76
  constraint parallel L75 L77
  constraint parallel L76 L78
  constraint coincident L79 P4
  constraint coincident L80 P4
  constraint midpoint L73 P4
  constraint coincident L1.end L2.start
  constraint coincident L4.start L5.end
  constraint coincident L4.end L7.end
  constraint coincident L0.end L1.start
  constraint horizontal L83
  constraint perpendicular L83 L84
  constraint parallel L83 L85
  constraint parallel L84 L86
  constraint coincident L87 P5
  constraint coincident L88 P5
  constraint midpoint L82 P5
  measures "d75" distance of P0 L20.end
  measures "d77" diameter of A1
  measures "d94" diameter of A3
  measures "d95" diameter of A4
  measures "d130" distance of L24.end P3
  measures "d132" distance of L23 L25
  measures "d133" distance of L27.start L29.end
  measures "d134" distance of L26.start L30.end
  measures "d135" distance of L26.start L32.end
  measures "d136" distance of L27.start L27.end
  measures "d137" distance of L33.start L33.end
  measures "d138" distance of L33.end L34.end
  measures "d139" distance of L38.end L36.start
  measures "d140" distance of L38.end L37.end
  measures "d141" distance of L24 L38
  measures "d178" distance of L76.end L77.end
  measures "d179" distance of L75.end L76.end
  measures "d180" distance of L84.end L85.end
  measures "d181" distance of L83.end L84.end
extrude "Extrude13" add sketch "Top Plate" along normal blind 3 separate body contours L0 L2 L3 L84 | L27 L28 L29 L30 L31 L32 L33 L34 L35 L36 L37 L38 L39 L40 L41 L42 L43 L44 L45 L46 L47 L48 L49 L50 L51 L52 L53 L54 L55 L56 L57 L58 L59 L60 L61 L62 L63 L64 L65 L66 L67 L68 L69 L70 L71 L72 makes body 7
extrude "Extrude14" add sketch "Top Plate" along normal blind 8 contours A3 | A4 bodies 7
extrude "Extrude15" add sketch "Top Plate" along normal blind 3 contours A1 | A2 bodies 7
sketch "Bottom Plate" plane through (42, 0, 0) normal (1, 0, 0) x (0, 1, 0)
  line L0 (8, 0) -> (0, 0)
  line L1 (0, 0) -> (0, -3)
  line L2 (0, -3) -> (8, -3)
  line L3 (8, -3) -> (8, 0)
  line L4 (-17, 52) -> (-17, 49)
  line L5 (-25, 49) -> (-17, 49)
  line L6 (-17.7031, 7) -> (-13.2642, 7)
  line L7 (28, 12) -> (28, 22)
  line L8 (-9, 49) -> (-9, 52)
  line L9 (-25, 30) -> (-28, 30)
  line L10 (-28, 12) -> (-28, 22)
  line L11 (25, 49) -> (25, 40)
  line L12 (25, 12) -> (-25, 12) construction
  line L13 (-8, -3) -> (-16, -3)
  line L14 (-8, 0) -> (-16, 0)
  line L15 (-28, -19) -> (-28, -9)
  line L16 (-9, -25) -> (-9, -28)
  line L17 (-25, -19) -> (-28, -19)
  line L18 (-8, -3) -> (-8, 0)
  line L19 (-9, -28) -> (-17, -28)
  line L20 (-25, -25) -> (-17, -25)
  line L21 (-16, 0) -> (-16, -3)
  line L22 (-8, 0) -> (-8, -3)
  line L23 (-25, -19) -> (-25, -25)
  line L24 (-9, -25) -> (0, -25)
  line L25 (-25, 12) -> (-28, 12)
  line L26 (-28, 22) -> (-25, 22)
  line L27 (17, 52) -> (17, 49)
  line L28 (9, 49) -> (0, 49)
  line L29 (25, 12) -> (25, -9)
  line L30 (-28, 30) -> (-28, 40)
  line L31 (28, 22) -> (25, 22)
  line L32 (0, 3.5) -> (0, 23.5) construction
  line L33 (28, 30) -> (28, 40)
  line L34 (-25, 49) -> (-25, 40)
  line L35 (-25, -25) -> (-25, 49) construction
  line L36 (25, 12) -> (28, 12)
  line L37 (28, 40) -> (25, 40)
  line L38 (0, 3.5) -> (25, 3.5) construction
  line L39 (9, 49) -> (9, 52)
  line L40 (9, 52) -> (17, 52)
  line L41 (25, 30) -> (28, 30)
  line L42 (-9, 49) -> (0, 49)
  line L43 (-28, 40) -> (-25, 40)
  line L44 (25, 30) -> (25, 22)
  line L45 (-25, 30) -> (-25, 22)
  line L46 (-9, 52) -> (-17, 52)
  line L47 (25, 49) -> (17, 49)
  line L48 (-25, 49) -> (25, 49) construction
  line L49 (25, -25) -> (17, -25)
  line L50 (25, -19) -> (25, -25)
  line L51 (25, -19) -> (28, -19)
  line L52 (16, -3) -> (8, -3)
  line L53 (-16, -3) -> (-8, -3)
  line L54 (-16, 0) -> (-16, -3)
  line L55 (-8, 0) -> (-16, 0)
  line L56 (-28, -9) -> (-25, -9)
  line L57 (-17, -28) -> (-17, -25)
  line L58 (17, -28) -> (17, -25)
  line L59 (25, 49) -> (25, -25) construction
  line L60 (16, -3) -> (16, 0)
  line L61 (9, -28) -> (17, -28)
  line L62 (9, -25) -> (9, -28)
  line L63 (-25, 12) -> (-25, -9)
  line L64 (28, -19) -> (28, -9)
  line L65 (0, 0) -> (-8, 0)
  line L66 (8, 0) -> (8, -3)
  line L67 (-8, -3) -> (0, -3)
  line L68 (28, -9) -> (25, -9)
  line L69 (8, -3) -> (16, -3)
  line L70 (0, -3) -> (0, 0)
  line L71 (-8, 0) -> (-8, -3)
  line L72 (9, -25) -> (0, -25)
  line L73 (8, 0) -> (16, 0)
  line L74 (16, 0) -> (16, -3)
  line L75 (16, 0) -> (8, 0)
  line L76 (8, 0) -> (8, -3)
  line L77 (16, -3) -> (8, 0) construction
  line L78 (8, -3) -> (16, 0) construction
  line L79 (-8, -3) -> (-16, 0) construction
  line L80 (-16, -3) -> (-8, 0) construction
  line L81 (7.75, -3.25) -> (16.25, -3.25)
  line L82 (16.25, -3.25) -> (16.25, 0.25)
  line L83 (16.25, 0.25) -> (7.75, 0.25)
  line L84 (7.75, 0.25) -> (7.75, -3.25)
  line L85 (7.75, -3.25) -> (16.25, 0.25) construction
  line L86 (16.25, -3.25) -> (7.75, 0.25) construction
  line L87 (-16.25, -3.25) -> (-7.75, -3.25)
  line L88 (-7.75, -3.25) -> (-7.75, 0.25)
  line L89 (-7.75, 0.25) -> (-16.25, 0.25)
  line L90 (-16.25, 0.25) -> (-16.25, -3.25)
  line L91 (-16.25, -3.25) -> (-7.75, 0.25) construction
  line L92 (-7.75, -3.25) -> (-16.25, 0.25) construction
  point P0 (-25, 3.5)
  point P1 (-25, -25)
  point P2 (-25, -25)
  point P3 (12, -1.5)
  point P4 (-12, -1.5)
  dimension "d142" = 20
  dimension "d146" = 50
  dimension "d147" = 42
  dimension "d148" = 10
  dimension "d149" = 3
  dimension "d150" = 10
  dimension "d151" = 3
  dimension "d152" = 3
  dimension "d153" = 10
  dimension "d154" = 8
  dimension "d155" = 3
  dimension "d156" = 8
  dimension "d182" = 8.5
  dimension "d183" = 3.5
  dimension "d184" = 8.5
  dimension "d185" = 3.5
  constraint vertical L32
  constraint vertical L35
  constraint horizontal L48
  constraint vertical L59
  constraint midpoint L12.start L59
  constraint midpoint L12.end L35
  constraint horizontal L51
  constraint vertical L64
  constraint horizontal L68
  constraint coincident L50.start L59
  constraint horizontal L36
  constraint vertical L7
  constraint horizontal L31
  constraint horizontal L41
  constraint vertical L33
  constraint horizontal L37
  constraint coincident L41.start L59
  constraint vertical L39
  constraint horizontal L40
  constraint vertical L27
  constraint coincident L27.end L48
  constraint midpoint L28.end L48
  constraint symmetric P0 L38.end L32
  constraint symmetric P2 L49.start L32
  constraint symmetric L5.start L11.start L32
  constraint symmetric L12.end L12.start L32
  constraint symmetric L17.start L50.start L32
  constraint symmetric L15.start L51.end L32
  constraint symmetric L15.end L64.end L32
  constraint symmetric L56.end L29.end L32
  constraint symmetric L10.start L7.start L32
  constraint symmetric L10.end L7.end L32
  constraint symmetric L26.end L31.end L32
  constraint symmetric L5.start P2 L12
  constraint symmetric L11.start L49.start L12
  constraint symmetric L49.end L27.end L12
  constraint symmetric L62.start L28.start L12
  constraint symmetric L61.start L39.end L12
  constraint symmetric L58.start L27.start L12
  constraint symmetric L28.end L24.end L12
  constraint symmetric L24.end L28.end L12
  constraint symmetric P2 L5.start L12
  constraint symmetric L19.end L4.start L12
  constraint symmetric L20.end L4.end L12
  constraint symmetric L16.start L8.start L12
  constraint symmetric L16.end L8.end L12
  constraint coincident P2 P1
  constraint coincident L12.end L25.start
  constraint coincident L24.end L72.end
  constraint coincident L49.start L50.end
  constraint parallel L35 L63
  constraint parallel L34 L57
  constraint parallel L24 L46
  constraint parallel L34 L45
  constraint vertical L38.end L49.start
  constraint equal L44 L65
  constraint parallel L77 L79
  constraint parallel L78 L80
  constraint horizontal L81
  constraint perpendicular L81 L82
  constraint parallel L81 L83
  constraint parallel L82 L84
  constraint coincident L85 P3
  constraint coincident L86 P3
  constraint midpoint L78 P3
  constraint horizontal L87
  constraint perpendicular L87 L88
  constraint parallel L87 L89
  constraint parallel L88 L90
  constraint coincident L91 P4
  constraint coincident L92 P4
  constraint midpoint L79 P4
  measures "d142" distance of L32.start L32.end
  measures "d146" distance of P2 L49.start
  measures "d147" distance of L6 L48
  measures "d148" distance of L29.end L50.start
  measures "d149" distance of L12.start L7.start
  measures "d150" distance of L12.start L31.end
  measures "d151" distance of L50.start L51.end
  measures "d152" distance of L33.start L41.start
  measures "d153" distance of L33.start L33.end
  measures "d154" distance of L28.start L27.end
  measures "d155" distance of L27.end L27.start
  measures "d156" distance of L27 L59
  measures "d182" distance of L82.end L83.end
  measures "d183" distance of L81.end L82.end
  measures "d184" distance of L88.end L89.end
  measures "d185" distance of L87.end L88.end
extrude "Extrude18" add sketch "Bottom Plate" along normal blind 3 separate body contours L0 L1 L2 L70 L84 | L1 L65 L67 L70 L88 | L4 L5 L7 L8 L9 L10 L11 L15 L16 L17 L19 L20 L23 L24 L25 L26 L27 L28 L29 L30 L31 L33 L34 L36 L37 L39 L40 L41 L42 L43 L44 L45 L46 L47 L49 L50 L51 L56 L57 L58 L61 L62 L63 L64 L68 L72 makes body 8
sketch "Motor Lifter" plane through (42, 0, 0) normal (-1, 0, 0) x (0, -1, 0)
  line L0 (-17, -28) -> (-9, -28)
  line L1 (-9, -28) -> (-9, -25)
  line L2 (-9, -25) -> (9, -25)
  line L3 (9, -25) -> (9, -28)
  line L4 (9, -28) -> (17, -28)
  line L5 (17, -28) -> (17, -25)
  line L6 (17, -25) -> (25, -25)
  line L7 (25, -25) -> (25, -19)
  line L8 (25, -19) -> (28, -19)
  line L9 (28, -19) -> (28, -9)
  line L10 (28, -9) -> (25, -9)
  line L11 (25, -9) -> (25, 12)
  line L12 (25, 12) -> (28, 12)
  line L13 (28, 12) -> (28, 22)
  line L14 (28, 22) -> (25, 22)
  line L15 (25, 22) -> (25, 30)
  line L16 (25, 30) -> (28, 30)
  line L17 (28, 30) -> (28, 40)
  line L18 (28, 40) -> (25, 40)
  line L19 (25, 40) -> (25, 49)
  line L20 (25, 49) -> (17, 49)
  line L21 (17, 49) -> (17, 52)
  line L22 (17, 52) -> (9, 52)
  line L23 (9, 52) -> (9, 49)
  line L24 (9, 49) -> (-9, 49)
  line L25 (-9, 49) -> (-9, 52)
  line L26 (-9, 52) -> (-17, 52)
  line L27 (-17, 52) -> (-17, 49)
  line L28 (-17, 49) -> (-25, 49)
  line L29 (-25, 49) -> (-25, 40)
  line L30 (-25, 40) -> (-28, 40)
  line L31 (-28, 40) -> (-28, 30)
  line L32 (-28, 30) -> (-25, 30)
  line L33 (-25, 30) -> (-25, 22)
  line L34 (-25, 22) -> (-28, 22)
  line L35 (-28, 22) -> (-28, 12)
  line L36 (-28, 12) -> (-25, 12)
  line L37 (-25, 12) -> (-25, -9)
  line L38 (-25, -9) -> (-28, -9)
  line L39 (-28, -9) -> (-28, -19)
  line L40 (-28, -19) -> (-25, -19)
  line L41 (-25, -19) -> (-25, -25)
  line L42 (-25, -25) -> (-17, -25)
  line L43 (-17, -25) -> (-17, -28)
  line L44 (-8, 0) -> (0, 0)
  line L45 (8, 0) -> (0, 0)
  line L46 (0, 0) -> (0, 34.5) construction
  line L47 (6.15, 47) -> (-6.15, 47)
  line L48 (-6.15, 47) -> (-6.15, 22)
  line L49 (-6.15, 22) -> (6.15, 22)
  line L50 (6.15, 22) -> (6.15, 47)
  line L51 (6.15, 47) -> (-6.15, 22) construction
  line L52 (-6.15, 47) -> (6.15, 22) construction
  line L53 (-6.15, 47) -> (-8.15, 47)
  line L54 (-8.15, 47) -> (-8.15, 22)
  line L55 (-8.15, 22) -> (-6.15, 22)
  line L56 (-6.15, 22) -> (-6.15, 47)
  line L57 (6.15, 47) -> (8.15, 47)
  line L58 (8.15, 47) -> (8.15, 22)
  line L59 (8.15, 22) -> (6.15, 22)
  line L60 (6.15, 22) -> (6.15, 47)
  line L61 (16.25, 0.25) -> (16.25, -3.25)
  line L62 (16.25, -3.25) -> (7.75, -3.25)
  line L63 (7.75, -3.25) -> (7.75, 0.25)
  line L64 (7.75, 0.25) -> (16.25, 0.25)
  line L65 (-7.75, 0.25) -> (-7.75, -3.25)
  line L66 (-7.75, -3.25) -> (-16.25, -3.25)
  line L67 (-16.25, -3.25) -> (-16.25, 0.25)
  line L68 (-16.25, 0.25) -> (-7.75, 0.25)
  point P0 (0, 34.5)
  dimension "d159" = 34.5
  dimension "d160" = 12.3
  dimension "d161" = 25
  dimension "d162" = 2
  dimension "d163" = 2
  dimension "d164" = 25
  constraint coincident L44.end L45.end
  constraint perpendicular L45 L46
  constraint horizontal L47
  constraint perpendicular L47 L48
  constraint parallel L47 L49
  constraint parallel L48 L50
  constraint coincident L51 P0
  constraint coincident L52 P0
  constraint coincident P0 L46.end
  constraint horizontal L53
  constraint vertical L54
  constraint horizontal L55
  constraint vertical L56
  constraint horizontal L57
  constraint vertical L58
  constraint horizontal L59
  constraint vertical L60
  measures "d159" distance of L44.end P0
  measures "d160" distance of L48.end L49.end
  measures "d161" distance of L47.end L48.end
  measures "d162" distance of L47.end L53.end
  measures "d163" distance of L47.start L57.end
  measures "d164" distance of L47.start L49.end
extrude "Extrude19" add sketch "Motor Lifter" along normal blind 8.5 contours L47 L48 L49 L50 L56 L60 bodies 8
extrude "Extrude20" add sketch "Motor Lifter" along normal blind 20.5 contours L50 L57 L58 L59 L60 | L48 L53 L54 L55 L56 bodies 8
sketch "Side Plate" plane through (0, 25, 0) normal (0, 1, 0) x (-1, 0, 0)
  line L0 (-10, 0) -> (-30, 0)
  line L1 (-30, 0) -> (-30, -3)
  line L2 (-30, -3) -> (-10, -3)
  line L3 (-10, -3) -> (-10, 0)
  line L4 (-42, 30) -> (-42, 40)
  line L5 (-42, 40) -> (-45, 40)
  line L6 (-45, 40) -> (-45, 30)
  line L7 (-45, 30) -> (-42, 30)
  line L8 (-42, 12) -> (-42, 22)
  line L9 (-42, 22) -> (-45, 22)
  line L10 (-45, 22) -> (-45, 12)
  line L11 (-45, 12) -> (-42, 12)
  line L12 (-42, -19) -> (-42, -9)
  line L13 (-42, -9) -> (-45, -9)
  line L14 (-45, -9) -> (-45, -19)
  line L15 (-45, -19) -> (-42, -19)
  line L16 (-30, 0) -> (-42, 0)
  line L17 (-42, 0) -> (-42, -3)
  line L18 (-42, -3) -> (-30, -3)
  line L19 (-30, -3) -> (-30, 0)
  line L20 (2, 0) -> (-10, 0)
  line L21 (-10, 0) -> (-10, -3)
  line L22 (-10, -3) -> (2, -3)
  line L23 (2, -3) -> (2, 0)
  line L24 (34, 0) -> (22, 0)
  line L25 (22, 0) -> (22, -3)
  line L26 (22, -3) -> (34, -3)
  line L27 (34, -3) -> (34, 0)
  line L28 (66, 0) -> (54, 0)
  line L29 (54, 0) -> (54, -3)
  line L30 (54, -3) -> (66, -3)
  line L31 (66, -3) -> (66, 0)
  line L32 (86, -9) -> (86, -19)
  line L33 (86, -19) -> (89, -19)
  line L34 (89, -19) -> (89, -9)
  line L35 (89, -9) -> (86, -9)
  line L36 (86, 22) -> (86, 12)
  line L37 (86, 12) -> (89, 12)
  line L38 (89, 12) -> (89, 22)
  line L39 (89, 22) -> (86, 22)
  line L40 (86, 40) -> (86, 30)
  line L41 (86, 30) -> (89, 30)
  line L42 (89, 30) -> (89, 40)
  line L43 (89, 40) -> (86, 40)
  line L44 (-42, 40) -> (-42, 49)
  line L45 (-42, 49) -> (-45, 49)
  line L46 (-45, 49) -> (-45, 40)
  line L47 (-45, 40) -> (-42, 40)
  line L48 (86, -19) -> (86, -25)
  line L49 (86, -25) -> (89, -25)
  line L50 (89, -25) -> (89, -19)
  line L51 (89, -19) -> (86, -19)
  line L52 (-45, 49) -> (89, 49)
  line L53 (89, 49) -> (89, -25)
  line L54 (89, -25) -> (-45, -25)
  line L55 (-45, -25) -> (-45, 49)
  constraint horizontal L52
  constraint vertical L53
  constraint horizontal L54
  constraint vertical L55
  constraint coincident L49.end L50.start
  constraint coincident L45.end L46.start
extrude "Extrude21" add sketch "Side Plate" along normal blind 3 separate body contours L0 L1 L2 L3 L19 L21 | L4 L7 L8 L9 L11 L12 L13 L15 L32 L35 L36 L37 L39 L40 L41 L43 L44 L48 L52 L53 L54 L55 | L5 L44 L45 L46 L47 L52 L55 | L33 L48 L49 L50 L51 L53 L54 makes body 9
mirror "Mirror1" about plane through (0, 0, 0) normal (0, 1, 0) of bodies 9 makes body 10
sketch "Connector Rod Clearance" plane through (0, 0, 12) normal (0, 0, 1) x (-1, 0, 0)
  circle A0 centre (-10, 0) radius 2
  circle A1 centre (30, 0) radius 2
  arc A2 (-10, 4) -> (-10, -4) centre (-10, 0) ccw
  line L0 (-10, -4) -> (30, -4)
  arc A3 (30, -4) -> (30, 4) centre (30, 0) ccw
  line L1 (30, 4) -> (-10, 4)
  circle A4 centre (-10, 0) radius 2
  circle A5 centre (30, 0) radius 2
  circle A6 centre (-10, 0) radius 2.15
  circle A7 centre (30, 0) radius 2.15
  dimension "d174" = 4.3
  dimension "d175" = 4.3
  constraint concentric A0 A6
  constraint concentric A1 A7
  measures "d174" diameter of A6
  measures "d175" diameter of A7
extrude "Extrude22" cut sketch "Connector Rod Clearance" against normal blind 5 contours A6 | A7 bodies 2
ref_plane "WorkPlane1" through (-30, 0, 12.5) normal (0, 0, 1) x (-1, 0, 0)
sketch "Sketch16" plane through (0, 0, 12.5) normal (0, 0, 1) x (1, 0, 0)
  circle A0 centre (-30, 0) radius 2
  circle A1 centre (-30, 0) radius 3
  circle A2 centre (10, 0) radius 2
  circle A3 centre (10, 0) radius 3
  dimension "d187" = 6
  dimension "d188" = 6
  constraint concentric A0 A1
  constraint concentric A2 A3
  measures "d187" diameter of A1
  measures "d188" diameter of A3
extrude "Extrude23" add sketch "Sketch16" along normal blind 4 separate body contours A0 | A1 | A2 | A3 makes body 11 at (-27.0149, -0.2987, 13.8333) makes body 12 at (12.9851, -0.2987, 13.8333)
extrude "Extrude24" cut sketch "Connector Rod Clearance" 2 faces at (9.427, 0.4727, 12) (-29.3851, 0.0994, 12) along normal blind 2 contours A6 | A7 on bodies 1 3 bodies 11 12
extrude "Extrude25" add sketch "Connector Rod Clearance" along normal blind 2 contours A0 A4 | A1 A5 bodies 1 3 4 7 8 9 10
equation "d1 = thickness"
equation "d3 = thickness"
equation "d16 = peg_diameter"
equation "screw_hole_diam = 3.5 mm"
equation "screw_inset = 2 mm"
equation "wing_movement = 20 mm"
equation "root_fillet = 1 mm"
equation "module = 3"
equation "d22 = screw_hole_diam"
equation "thickness = 7 mm"
equation "inset_diameter = 7 mm"
equation "d25 = inset_diameter"
equation "peg_diameter = 4 mm"
equation "d28 = peg_diameter"
equation "d29 = connector_thickness"
equation "d31 = -screw_inset"
equation "d35 = -thickness"
equation "d37 = -thickness"
equation "connector_thickness = 5 mm"
equation "d40 = connector_thickness"
equation "d42 = connector_thickness"
equation "d44 = dowel_hole_diameter"
equation "d45 = thickness / 2"
equation "d49 = base_width"
equation "d52 = backing_screw_hole_diam"
equation "d53 = backing_screw_hole_diam"
equation "d55 = slider_clearence"
equation "slider_clearence = 0.3 mm"
equation "d60 = thickness - slider_clearence"
equation "d71 = 128 / 32"
equation "d73 = 128 mm - 32 mm"
equation "dowel_hole_diameter = 5.5 mm"
equation "d77 = dowel_hole_diameter"
equation "dowel_hole_wall = 2 mm"
equation "base_width = 50 mm"
equation "base_height = 128 mm"
equation "base_length = 80 mm"